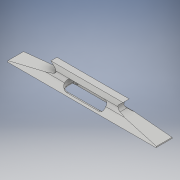
# Autodesk Inventor part: koma
Saved by Autodesk Inventor 2019 (Build 230136000, 136)
## iProperties
Created: 2019-12-27
Part Number: koma
Material: Типовые
Document SubType Name: Modeling
Designer: stepa
Density: 1 g/cm^3
Appearance: По умолчанию
Author: stepa
Autodesk Inventor part; units mm, degrees
ref_plane "YZ Plane" through (0, 0, 0) normal (1, 0, 0) x (0, 1, 0)
ref_plane "XZ Plane" through (0, 0, 0) normal (0, 1, 0) x (-1, 0, 0)
ref_plane "XY Plane" through (0, 0, 0) normal (0, 0, 1) x (1, 0, 0)
sketch "Эскиз1" plane through (0, 0, 0) normal (0, 1, 0) x (-1, 0, 0)
  line L0 (0, 0) -> (-72, 0)
  line L1 (-72, 0) -> (-72, -8)
  line L2 (-72, -8) -> (0, -8)
  line L3 (0, -8) -> (0, 0)
  dimension "d0" = 72
  dimension "d1" = 8
  constraints: 8 end point, 2 parallel, 1 horizontal, 1 perpendicular
  measures "d0" distance of L2.end L1.end
  measures "d1" distance of L1.end L0.end
extrude "Выдавливание1" add sketch "Эскиз1" along normal blind 8.5
sketch "Эскиз2" plane through (0, 0, 0) normal (0, 0, 1) x (1, 0, 0)
  line L0 (0, 0) -> (72, 0) projected
  line L1 (72, 0) -> (72, 8.5) projected
  line L2 (0, 8.5) -> (72, 8.5) projected
  line L3 (0, 0) -> (0, 8.5) projected
  line L4 (0, 0) -> (0, 8.5) projected
  line L5 (0, 0.5) -> (19.7616, 4)
  line L6 (72, 0.5) -> (52.2384, 4)
  arc A0 (19.7616, 4) -> (20.5343, 6.5634) centre (19.5, 5.477) ccw
  arc A1 (51.4657, 6.5634) -> (52.2384, 4) centre (52.5, 5.477) ccw
  line L7 (20.5343, 6.5634) -> (18.5, 8.5)
  line L8 (51.4657, 6.5634) -> (53.5, 8.5)
  line L9 (28.25, 1) -> (43.75, 1)
  line L10 (28.25, 5.5) -> (43.75, 5.5)
  arc A2 (28.25, 5.5) -> (28.25, 1) centre (28.25, 3.25) ccw
  arc A3 (43.75, 1) -> (43.75, 5.5) centre (43.75, 3.25) ccw
  line L11 (0, 8.5) -> (72, 8.5) projected
  line L12 (18.5, 8.5) -> (53.5, 8.5)
  line L13 (0, 0.5) -> (0, 0)
  line L14 (0, 0) -> (72, 0) projected
  line L15 (0, 0) -> (72, 0)
  line L16 (72, 0) -> (72, 0.5)
  dimension "d4" = 0.5
  dimension "d5" = 4
  dimension "d7" = 33
  dimension "d12" = 1.5
  dimension "d13" = 1
  dimension "d14" = 3
  dimension "d15" = 2.25
  dimension "d16" = 8.75
  dimension "d18" = 8.75
  dimension "d19" = 35
  constraints: 20 end point, 8 point on circle, 6 tangent, 4 centre point, 4 horizontal, 4 horizontal alignment, 3 equal length, 3 point on line, 2 perpendicular, 1 equal radius, 1 vertical alignment
  measures "d4" distance from line of L6.start L0
  measures "d5" distance from line of L0 L5.end
  measures "d7" distance of A1.centre A0.centre
  measures "d12" radius of A0
  measures "d13" distance between parallel lines of L9 L0
  measures "d14" distance between parallel lines of L2 L10
  measures "d15" radius of A2
  measures "d16" horizontal distance of A2.centre A0.centre
  measures "d18" horizontal distance of A1.centre A3.centre
  measures "d19" distance of L7.end L8.end
extrude "Выдавливание2" cut sketch "Эскиз2" against normal through all contours L3 L5 A0 L7 L2 L8 A1 L6 L1 L0 keep common part
sketch "Эскиз3" plane through (72, 0, 0) normal (1, 0, 0) x (0, 0, -1)
  line L0 (8, 0) -> (8, 0.5) projected
  line L1 (8, 0.5) -> (8, 4) projected
  line L2 (0, 0) -> (8, 0) projected
  line L3 (0, 0) -> (0, 0.5) projected
  line L4 (0, 4) -> (0, 0.5) projected
  line L5 (0, 6.5634) -> (0, 4) projected
  line L6 (0, 8.5) -> (0, 6.5634) projected
  line L7 (8, 8.5) -> (0, 8.5) projected
  line L8 (8, 6.5634) -> (8, 8.5) projected
  line L9 (8, 4) -> (8, 6.5634) projected
  line L10 (0, 5.5) -> (8, 5.5) projected
  line L11 (2.5, 8.5) -> (2.5, 5.5)
  line L12 (5.5, 8.5) -> (5.5, 5.5)
  line L13 (0, 5.5) -> (0, 1) projected
  line L14 (2.5, 8.5) -> (5.5, 8.5)
  line L15 (0, 0) -> (2.5, 5.5)
  line L16 (8, 0) -> (5.5, 5.5)
  line L17 (0, 0) -> (8, 0)
  point P0 (4, 8.5)
  point P1 (4, 8.5)
  dimension "d22" = 3
  constraints: 12 end point, 4 point on line, 2 midpoint, 1 coincident, 1 collinear, 1 horizontal, 1 perpendicular, 1 vertical
  measures "d22" distance between parallel lines of L12 L11
extrude "Выдавливание3" cut sketch "Эскиз3" against normal through all contours L2 L15 L10 L16 | L10 L11 L7 L12 keep common part
sketch "Эскиз4" plane through (72, 0, 0) normal (1, 0, 0) x (0, 0, -1)
  line L0 (2.5, 6.5634) -> (2.5, 8.5) projected
  line L1 (5.5, 8.5) -> (2.5, 8.5) projected
  line L2 (5.5, 8.5) -> (5.5, 6.5634) projected
  line L3 (5.5, 6.5634) -> (5.5, 5.5) projected
  line L4 (2.5, 5.5) -> (2.5, 6.5634) projected
  line L5 (1.8182, 4) -> (2.5, 5.5) projected
  line L6 (5.5, 5.5) -> (6.1818, 4) projected
  line L7 (6.1818, 4) -> (7.7727, 0.5) projected
  line L8 (0.2273, 0.5) -> (1.8182, 4) projected
  line L9 (0, 0) -> (0.2273, 0.5) projected
  line L10 (7.7727, 0.5) -> (8, 0) projected
  line L11 (2.5, 5.5) -> (5.5, 5.5) projected
  arc A0 (1.5909, 3.5) -> (2.5, 5.5) centre (1.1155, 4.9227) ccw
  arc A1 (5.5, 5.5) -> (6.4091, 3.5) centre (6.8845, 4.9227) ccw
  line L12 (0.4545, 1) -> (2.5, 5.5) projected
  line L13 (2.5, 5.5) -> (5.5, 5.5) projected
  line L14 (0.4545, 1) -> (7.5455, 1) projected
  line L15 (1.8182, 4) -> (2.5, 5.5) projected
  line L16 (2.5, 5.5) -> (1.5909, 3.5)
  line L17 (5.5, 5.5) -> (6.4091, 3.5)
  line L18 (5.5, 5.5) -> (7.5455, 1) projected
  dimension "d25" = 1.5
  dimension "d26" = 1.5
  dimension "d27" = 2
  constraints: 4 end point, 4 point on circle, 2 centre point, 2 collinear, 2 point on line, 1 equal radius, 1 horizontal alignment
  measures "d25" radius of A0
  measures "d26" vertical distance of L4.start L5.start
  measures "d27" vertical distance of L16.end L4.start
extrude "Выдавливание4" cut sketch "Эскиз4" against normal through all contours A0 L8 L5 | L6 L7 A1
sketch "Эскиз5" plane through (0, 0, 0) normal (0, -1, 0) x (1, 0, 0)
  line L0 (26, -1.4773) -> (26, -6.5227) projected
  line L1 (46, -1.4773) -> (46, -6.5227) projected
  line L2 (0, 0) -> (72, 0) projected
  line L3 (0, -8) -> (0, 0) projected
  line L4 (72, -8) -> (0, -8) projected
  line L5 (72, 0) -> (72, -8) projected
  line L6 (26, -1) -> (46, -1)
  line L7 (46, -1) -> (46, -7)
  line L8 (46, -7) -> (26, -7)
  line L9 (26, -7) -> (26, -1)
  dimension "d30" = 1
  dimension "d31" = 1
  constraints: 8 end point, 2 collinear, 2 parallel, 1 horizontal, 1 perpendicular
  measures "d30" distance between parallel lines of L2 L6
  measures "d31" distance between parallel lines of L4 L8
extrude "Выдавливание5" cut sketch "Эскиз5" against normal blind 1.3 contours L9 L6 L7 L1 L8 L0
sketch "Эскиз6" plane through (0, 0, 0) normal (0, -1, 0) x (1, 0, 0)
  line L0 (26, -7) -> (26, -1) projected
  line L1 (26, -1) -> (46, -1) projected
  line L2 (46, -1) -> (46, -7) projected
  line L3 (46, -7) -> (26, -7) projected
  line L4 (0, 0) -> (72, 0) projected
  line L5 (0, -8) -> (0, 0) projected
  line L6 (72, -8) -> (0, -8) projected
  line L7 (72, 0) -> (72, -8) projected
  line L8 (5, -4) -> (26, -1)
  line L9 (5, -4) -> (26, -7)
  line L10 (67, -4) -> (46, -1)
  line L11 (67, -4) -> (46, -7)
  point P0 (72, -4)
  dimension "d34" = 5
  dimension "d35" = 5
  constraints: 8 end point, 2 horizontal alignment, 1 midpoint
  measures "d34" distance from line of L8.start L5
  measures "d35" distance of point (72, -4) L10.start
extrude "Выдавливание6" cut sketch "Эскиз6" against normal blind 1.3 contours L9 L8 L0 | L2 L10 L11
fillet "Сопряжение1" radius 1.3 4 edges at (15.5, 1.3, -5.5) (15.5, 1.3, -2.5) (56.5, 1.3, -2.5) (56.5, 1.3, -5.5)
fillet "Сопряжение2" radius 0.5 10 edges at (27.4777, 1.1367, -6.5351) (28.7844, 1, -6.9237) (27.4777, 1.1367, -1.4649) (28.7844, 1, -1.0763) (27.1275, 1.3, -4) (44.5219, 1.1366, -1.4646) (43.2156, 1, -1.0763) (44.5219, 1.1366, -6.5354) (43.2156, 1, -6.9237) (44.8725, 1.3, -4)
equation "\"d18\" = d16"
